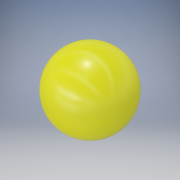
# Autodesk Inventor part: Tennis Ball
Saved by Autodesk Inventor 2019 (Build 230136000, 136)
## iProperties
Created: 2019-01-29
Part Number: Tennis Ball
Material: Generic
Document SubType Name: Modeling
Designer: Varga Daniel
Density: 1 g/cm^3
Appearance: Yellow
Author: Varga Daniel
Autodesk Inventor part; units mm, degrees
ref_plane "YZ Plane" through (0, 0, 0) normal (1, 0, 0) x (0, 1, 0)
ref_plane "XZ Plane" through (0, 0, 0) normal (0, 1, 0) x (-1, 0, 0)
ref_plane "XY Plane" through (0, 0, 0) normal (0, 0, 1) x (1, 0, 0)
sketch "Sketch1" plane through (0, 0, 0) normal (0, 0, 1) x (1, 0, 0)
  arc A0 (0, -33.5) -> (0, 33.5) centre (0, 0) ccw
  line L0 (0, 33.5) -> (0, -33.5)
  dimension "d0" = 67
  constraints: 2 end point, 2 point on circle, 1 centre point, 1 coincident, 1 midpoint, 1 vertical
  measures "d0" diameter of A0
revolve "Revolution1" add sketch "Sketch1" angle 360 about axis through (0, 33.5, 0) along (0, -1, 0)
body "Solid1"
